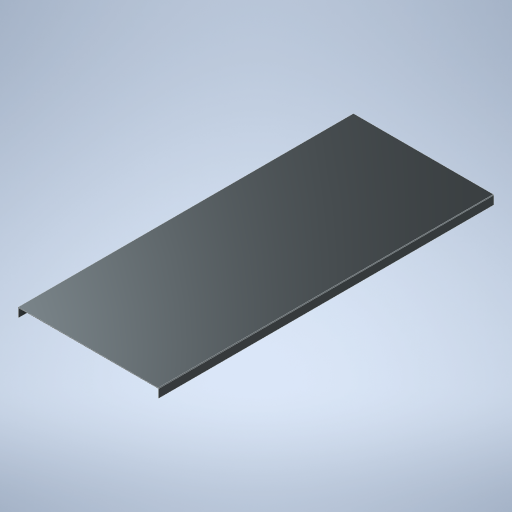
# Autodesk Inventor part: IronFrame
Saved by Autodesk Inventor 2023 (Build 270158000, 158)
## iProperties
Created: 2022-10-13
Part Number: IronFrame
Material: Iron, Cast
Document SubType Name: Modeling
Designer: mliu-23
Density: 7.15 g/cm^3
Appearance: Iron Gray
Author: mliu-23
Autodesk Inventor part; units mm, degrees
ref_plane "YZ Plane" through (0, 0, 0) normal (1, 0, 0) x (0, 1, 0)
ref_plane "XZ Plane" through (0, 0, 0) normal (0, 1, 0) x (-1, 0, 0)
ref_plane "XY Plane" through (0, 0, 0) normal (0, 0, 1) x (1, 0, 0)
sketch "Sketch1" plane through (0, 0, 0) normal (0, 1, 0) x (-1, 0, 0)
  line L0 (-425.45, 1016) -> (425.45, 1016)
  line L1 (425.45, 1016) -> (425.45, -1016)
  line L2 (425.45, -1016) -> (-425.45, -1016)
  line L3 (-425.45, -1016) -> (-425.45, 1016)
  line L4 (-425.45, 1016) -> (425.45, -1016) construction
  line L5 (425.45, 1016) -> (-425.45, -1016) construction
  point P0 (0, 0)
  dimension "d0" = 850.9
  dimension "d1" = 2032
  constraints: 12 end point, 2 midpoint, 2 parallel, 1 horizontal, 1 perpendicular
  measures "d0" distance of L1.end L2.end
  measures "d1" distance of L0.end L1.end
extrude "Extrusion1" add sketch "Sketch1" along normal blind 3.175
sketch "Sketch2" plane through (0, 0, 0) normal (0, -1, 0) x (1, 0, 0)
  line L0 (425.45, -1016) -> (-425.45, -1016) projected
  line L1 (425.45, 1016) -> (425.45, -1016) projected
  line L2 (-425.45, 1016) -> (425.45, 1016) projected
  line L3 (-425.45, -1016) -> (-425.45, 1016) projected
  line L4 (-425.45, 1016) -> (425.45, 1016) projected
  line L5 (425.45, -1016) -> (-425.45, -1016) projected
  line L6 (425.45, 1016) -> (422.275, 1016)
  line L7 (422.275, 1016) -> (422.275, -1016)
  line L8 (422.275, -1016) -> (425.45, -1016)
  line L9 (425.45, -1016) -> (425.45, 1016)
  line L10 (-425.45, -1016) -> (-425.45, 1016) projected
  line L11 (-425.45, 1016) -> (-422.275, 1016)
  line L12 (-422.275, 1016) -> (-422.275, -1016)
  line L13 (-422.275, -1016) -> (-425.45, -1016)
  line L14 (-425.45, -1016) -> (-425.45, 1016)
  point P0 (0, 0)
  dimension "d4" = 3.175
  dimension "d5" = 3.175
  constraints: 16 end point, 4 parallel, 2 horizontal, 2 perpendicular, 2 point on line
  measures "d4" distance of L11.end L2.start
  measures "d5" distance between parallel lines of L1 L7
extrude "Extrusion2" add sketch "Sketch2" along normal blind 50.8 contours L0 L7 L2 L1 | L0 L3 L2 L12
fillet "Fillet1" radius 3.175 2 edges at (-422.275, 0, 0) (425.45, 3.175, 0)
body "Solid1"
